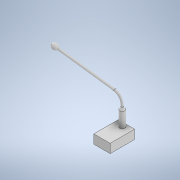
# Autodesk Inventor part: 無線麥克風組
Saved by Autodesk Inventor 2021 (Build 250183000, 183)
## iProperties
Created: 2023-02-19
Part Number: 無線麥克風組
Material: 一般
Document SubType Name: Modeling
Designer: brian
Density: 1 g/cm^3
Appearance: 預設
Author: brian
Autodesk Inventor part; units mm, degrees
ref_plane "YZ Plane" through (0, 0, 0) normal (1, 0, 0) x (0, 1, 0)
ref_plane "XZ Plane" through (0, 0, 0) normal (0, 1, 0) x (-1, 0, 0)
ref_plane "XY Plane" through (0, 0, 0) normal (0, 0, 1) x (1, 0, 0)
sketch "草圖1" plane through (0, 0, 0) normal (0, 1, 0) x (-1, 0, 0)
  line L0 (-50, 75) -> (50, 75)
  line L1 (50, 75) -> (50, -75)
  line L2 (50, -75) -> (-50, -75)
  line L3 (-50, -75) -> (-50, 75)
  line L4 (-50, 75) -> (50, -75) construction
  line L5 (50, 75) -> (-50, -75) construction
  point P0 (0, 0)
  dimension "d0" = 100
  dimension "d1" = 150
  constraints: 12 end point, 2 midpoint, 2 parallel, 1 horizontal, 1 perpendicular
  measures "d0" distance of L1.end L2.end
  measures "d1" distance of L0.end L1.end
extrude "擠出1" add sketch "草圖1" along normal blind 55
sketch "草圖2" plane through (0, 55, 0) normal (0, 1, 0) x (1, 0, 0)
  circle A0 centre (0, 49.596879) radius 15.361397
  point P0 (0, 0)
  constraints: 1 centre point
extrude "擠出2" add sketch "草圖2" along normal blind 92.5
sketch "草圖3" plane through (0, 147.5, -49.596879) normal (0, 1, 0) x (1, 0, 0)
  circle A0 centre (0, 0) radius 15.361397
  point P0 (0, -49.596879)
extrude "擠出3" add sketch "草圖3" along normal blind 15 draft -30
sketch "草圖8" plane through (0, 162.5, -49.596879) normal (0, 1, 0) x (1, 0, 0)
  circle A0 centre (0, 0) radius 6.701143
  line L0 (0, 0) -> (-74.851571, -205.653002)
  line L1 (0, 0) -> (218.851354, 0) construction
  point P0 (0, -49.596879)
  dimension "d14" = 110
  constraints: 4 end point, 1 equal length, 1 horizontal
  measures "d14" angle of L0 L1
surface extrude "擠出表面2" sketch "草圖8" along normal blind 8 shown no curves L0
sketch "草圖4" plane through (-14.690503, 0, -9.235054) normal (0.9396926, 0, 0.3420201) x (0, 1, 0)
  line L0 (55, -69.985594) -> (0, -69.985594) construction
  line L1 (0, -69.985594) -> (0, 89.641072) construction
  line L2 (55, 89.641072) -> (55, -27.590761) construction
  line L3 (55, -27.590761) -> (147.5, -27.590761) construction
  line L4 (147.5, -27.590761) -> (162.5, -36.251015) construction
  line L5 (162.5, -36.251015) -> (162.5, -49.6533) construction
  line L6 (162.5, -49.6533) -> (147.5, -58.313554) construction
  line L7 (147.5, -58.313554) -> (55, -58.313554) construction
  line L8 (55, -58.313554) -> (55, -69.985594) construction
  line L9 (162.5, -36.251015) -> (162.5, -49.6533) construction
  arc A0 (162.5, -42.952157) -> (266.230331, -3.041729) centre (162.5, 111.804689) ccw
  line L10 (266.230331, -3.041729) -> (563.073853, 265.070045)
  line L11 (0, 89.641072) -> (55, 89.641072)
  point P0 (0, 3.653664)
  dimension "d8" = 400
  constraints: 2 end point, 2 point on circle, 1 centre point, 1 line through centre, 1 midpoint, 1 tangent
  measures "d8" distance of L10.start L10.end
sketch "草圖5" plane through (0, 162.5, -49.596879) normal (0, 1, 0) x (1, 0, 0)
  circle A0 centre (0, 0) radius 6.701143
  point P0 (0, -49.596879)
sweep "掃掠1" add profiles "草圖5" path "草圖4" path curves A0 L10
sketch "草圖6" plane through (-105.349798, 563.073853, 239.849311) normal (-0.2292491, 0.7421088, 0.6298566) x (0.9554499, 0.2951535, 0)
  circle A0 centre (0, 0) radius 6.701143
  circle A1 centre (0, 0) radius 6.701143
  line L0 (-6.701143, 0) -> (6.701143, 0)
  point P0 (-65.536753, -172.147129)
  point P1 (0, 0)
  constraints: 2 end point, 2 horizontal alignment, 2 point on circle, 1 midpoint
surface extrude "擠出表面1" sketch "草圖6" along normal blind 8 shown yes curves L0
sketch "草圖7" plane through (-98.947192, 565.051719, 239.849311) normal (-0.1859044, 0.6017964, -0.7767114) x (-0.9554499, -0.2951535, 0)
  line L0 (13.402285, 0) -> (0, 0)
  line L1 (13.402285, 0) -> (0, 0)
  spline S0 degree 4 poles (13.402285, 0) (44.904659, 17.87413) (4.281315, 87.58342) (-27.060021, 18.156606) (0, 0) knots 0 0 0 0 0 1 1 1 1 1
  line L2 (6.701143, 41.850443) -> (6.701143, 0)
  line L3 (13.402285, 0) -> (0, 0)
  point P0 (72.237896, -593.084089)
  point P1 (21.56931, 30.293196)
  point P2 (-7.261182, 30.293196)
  constraints: 2 end point, 1 horizontal alignment, 1 midpoint, 1 perpendicular, 1 vertical alignment, 5 other
revolve "迴轉1" add sketch "草圖7" angle 360 about axis through (-114.943973, 594.131436, 266.20909) along (0.2292491, -0.7421088, -0.6298566) picked at (11.989428, 23.179775) contours L0 L2 S0
body "Srf1"
body "Srf2"
